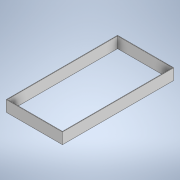
# Autodesk Inventor part: vib_bed_full_xz
Saved by Autodesk Inventor 2021 (Build 250183000, 183)
## iProperties
Created: 2020-07-18
Part Number: vib_bed_full_xz
Material: Generic
Document SubType Name: Modeling
Designer: dwer2
Density: 1 g/cm^3
Appearance: Default
Author: dwer2
Autodesk Inventor part; units mm, degrees
ref_plane "YZ Plane" through (0, 0, 0) normal (1, 0, 0) x (0, 1, 0)
ref_plane "XZ Plane" through (0, 0, 0) normal (0, 1, 0) x (-1, 0, 0)
ref_plane "XY Plane" through (0, 0, 0) normal (0, 0, 1) x (1, 0, 0)
sketch "Sketch2" plane through (0, 0, 0) normal (0, 1, 0) x (-1, 0, 0)
  line L0 (0, 0) -> (-20, 0) projected
  line L1 (0, 0) -> (100, 0)
  line L2 (100, 0) -> (100, 200)
  line L3 (100, 200) -> (0, 200)
  line L4 (0, 200) -> (0, 0)
  line L5 (101, 201) -> (-1, 201)
  line L6 (-1, 201) -> (-1, -1)
  line L7 (-1, -1) -> (101, -1)
  line L8 (101, -1) -> (101, 201)
  dimension "d8" = 100
  dimension "d9" = 200
  dimension "d10" = 1
  dimension "d11" = 1
  dimension "d12" = 1
  dimension "d13" = 1
  constraints: 16 end point, 4 parallel, 2 horizontal, 2 perpendicular
  measures "d8" distance of L2.end L3.end
  measures "d9" distance of L1.end L2.end
  measures "d10" distance between parallel lines of L2 L8
  measures "d11" distance between parallel lines of L1 L7
  measures "d12" distance between parallel lines of L4 L6
  measures "d13" distance between parallel lines of L3 L5
extrude "Extrusion2" add sketch "Sketch2" along normal blind 20
equation "\"d8\" = inner_width"
equation "\"d9\" = height"
equation "\"d10\" = wall_thicknes"
equation "\"d11\" = wall_thicknes"
equation "\"d12\" = wall_thicknes"
equation "\"d13\" = wall_thicknes"
equation "\"inner_width\" = 100"
equation "\"height\" = 200"
equation "\"wall_thicknes\" = 1"
body "Solid2"
